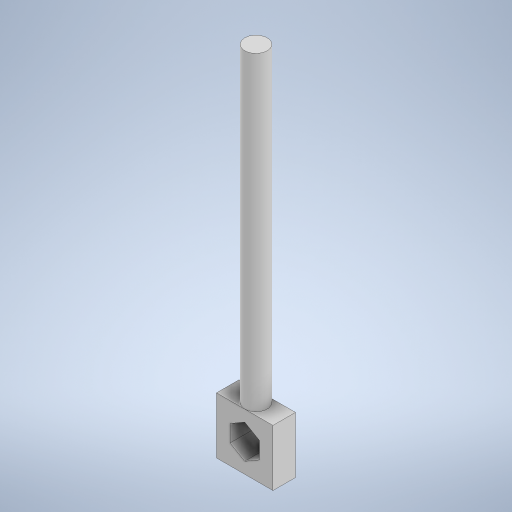
# Autodesk Inventor part: dźwignia
Saved by Autodesk Inventor 2024 (Build 280153000, 153)
## iProperties
Created: 2024-09-17
Part Number: dźwignia
Material: Ogólny
Document SubType Name: Modeling
Designer: JEDEN
Density: 1 g/cm^3
Appearance: Domyślna
Author: JEDEN
Autodesk Inventor part; units mm, degrees
ref_plane "YZ Plane" through (0, 0, 0) normal (1, 0, 0) x (0, 1, 0)
ref_plane "XZ Plane" through (0, 0, 0) normal (0, 1, 0) x (-1, 0, 0)
ref_plane "XY Plane" through (0, 0, 0) normal (0, 0, 1) x (1, 0, 0)
sketch "Szkic1" plane through (0, 0, 0) normal (0, 0, 1) x (1, 0, 0)
  circle A0 centre (-8.3785, -3.5136) radius 15
  line L0 (-8.3785, 11.4864) -> (4.6118, 3.9864)
  line L1 (4.6118, 3.9864) -> (4.6118, -11.0136)
  line L2 (4.6118, -11.0136) -> (-8.3785, -18.5136)
  line L3 (-8.3785, -18.5136) -> (-21.3689, -11.0136)
  line L4 (-21.3689, -11.0136) -> (-21.3689, 3.9864)
  line L5 (-21.3689, 3.9864) -> (-8.3785, 11.4864)
  line L6 (-33.3785, 21.4864) -> (16.6215, 21.4864)
  line L7 (16.6215, 21.4864) -> (16.6215, -28.5136)
  line L8 (16.6215, -28.5136) -> (-33.3785, -28.5136)
  line L9 (-33.3785, -28.5136) -> (-33.3785, 21.4864)
  line L10 (-33.3785, 21.4864) -> (16.6215, -28.5136) construction
  line L11 (16.6215, 21.4864) -> (-33.3785, -28.5136) construction
  point P0 (0, 0)
  point P1 (-16.899, -8.3685)
  point P2 (-21.3689, 3.9864)
  dimension "d2" = 360
  dimension "d3" = 50
  dimension "d4" = 50
  constraints: 24 end point, 5 parallel, 2 midpoint, 2 point on circle, 1 centre point, 1 coincident, 1 horizontal, 1 perpendicular, 1 vertical, 7 other
  measures "d3" distance of L7.end L8.end
  measures "d4" distance of L6.end L7.end
extrude "Wyciągnięcie proste1" add sketch "Szkic1" along normal blind 20 contours A0 L1 | L0 A0 | A0 L2 | L5 A0 | A0 L3 | L4 A0 | L6 L7 L8 L9
sketch "Szkic2" plane through (-33.3785, 21.4864, 0) normal (0, 1, 0) x (1, 0, 0)
  line L0 (25, 0) -> (25, -20) projected
  circle A0 centre (25, -10) radius 10
  point P0 (33.3785, 0)
  dimension "d7" = 20
  constraints: 1 centre point, 1 coincident, 1 midpoint
  measures "d7" diameter of A0
extrude "Wyciągnięcie proste2" add sketch "Szkic2" along normal blind 275
